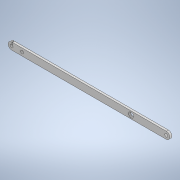
# Autodesk Inventor part: 零件2
Saved by Autodesk Inventor 2022.3 (Build 263350000, 350)
## iProperties
Created: 2023-04-16
Part Number: 零件2
Material: 一般
Document SubType Name: Modeling
Designer: JOU
Density: 1 g/cm^3
Appearance: 預設
Author: JOU
Autodesk Inventor part; units mm, degrees
ref_plane "YZ Plane" through (0, 0, 0) normal (1, 0, 0) x (0, 1, 0)
ref_plane "XZ Plane" through (0, 0, 0) normal (0, 1, 0) x (-1, 0, 0)
ref_plane "XY Plane" through (0, 0, 0) normal (0, 0, 1) x (1, 0, 0)
sketch "草圖1" plane through (0, 0, 0) normal (0, 0, 1) x (1, 0, 0)
  line L0 (-223.1596, 56.676) -> (-3.1596, 56.676) construction
  line L1 (-223.1596, 51.676) -> (-3.1596, 51.676)
  line L2 (-3.1596, 61.676) -> (-223.1596, 61.676)
  arc A0 (-223.1596, 61.676) -> (-223.1596, 51.676) centre (-223.1596, 56.676) ccw
  arc A1 (-3.1596, 51.676) -> (-3.1596, 61.676) centre (-3.1596, 56.676) ccw
  circle A2 centre (-223.1596, 56.676) radius 2.1
  circle A3 centre (-3.1596, 56.676) radius 2.1
  circle A4 centre (-208.1596, 56.676) radius 2.1
  circle A5 centre (-53.1596, 56.676) radius 3.5
  line L3 (-223.1596, 61.676) -> (-222.1596, 61.676)
  line L4 (-222.1596, 61.676) -> (-222.1596, 58.5227)
  line L5 (-222.1596, 58.5227) -> (-223.1596, 58.5227)
  line L6 (-223.1596, 58.5227) -> (-223.1596, 61.676)
  point P0 (0, 0)
  point P1 (-113.1596, 56.676)
  point P2 (-223.1596, 58.776)
  dimension "d2" = 4.2
  dimension "d0" = 220
  dimension "d1" = 10
  dimension "d3" = 4.2
  dimension "d4" = 4.2
  dimension "d5" = 15
  dimension "d8" = 7
  dimension "d9" = 50
  dimension "d10" = 1
  constraints: 16 end point, 5 centre point, 4 point on circle, 4 tangent, 3 parallel, 2 coincident, 2 horizontal, 2 point on line, 1 midpoint, 1 perpendicular, 3 other
  measures "d0" distance of L2.start L2.end
  measures "d1" distance between parallel lines of L1 L2
  measures "d3" diameter of A3
  measures "d4" diameter of A4
  measures "d5" distance of A4.centre point (-223.16, 56.676)
  measures "d8" diameter of A5
  measures "d9" distance of L0.end A5.centre
  measures "d10" distance of L4.end L5.end
extrude "擠出1" add sketch "草圖1" along normal blind 3 contours A0 L6 A2 L4 L2 A1 L1
